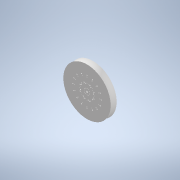
# Autodesk Inventor part: CenterIndexerWheel
Saved by Autodesk Inventor 2020 (Build 240168000, 168)
## iProperties
Created: 2020-01-19
Part Number: CenterIndexerWheel
Material: Generic
Document SubType Name: Modeling
Designer: srini
Density: 1 g/cm^3
Appearance: Default
Author: srini
Autodesk Inventor part; units mm, degrees
ref_plane "YZ Plane" through (0, 0, 0) normal (1, 0, 0) x (0, 1, 0)
ref_plane "XZ Plane" through (0, 0, 0) normal (0, 1, 0) x (-1, 0, 0)
ref_plane "XY Plane" through (0, 0, 0) normal (0, 0, 1) x (1, 0, 0)
sketch "Sketch1" plane through (0, 0, 0) normal (0, 0, 1) x (1, 0, 0)
  circle A0 centre (0, 0) radius 203.2
  dimension "d0" = 406.4
  constraints: 1 centre point, 1 coincident
  measures "d0" diameter of A0
extrude "Extrusion1" add sketch "Sketch1" along normal blind 50.8
sketch "Sketch2" plane through (0, 0, 0) normal (1, 0, 0) x (0, 1, 0)
  circle A0 centre (-285.75, 25.4) radius 88.9
  line L0 (203.2, 0) -> (-203.2, 0) projected
  line L1 (0, 149.86) -> (0, -99.06) projected
  point P0 (0, 0)
  dimension "d3" = 25.4
  dimension "d4" = 177.8
  dimension "d5" = 285.75
  constraints: 1 centre point
  measures "d3" distance from line of L0 A0.centre
  measures "d4" diameter of A0
  measures "d5" distance from line of L1 A0.centre
revolve "Revolution1" cut sketch "Sketch2" angle 360 about axis through (0, 0, 0) along (0, 0, -1)
sketch "Sketch3" plane through (0, 0, 0) normal (0, 0, -1) x (-1, 0, 0)
  point P0 (0, 0)
sketch "Sketch4" plane through (0, 0, 50.8) normal (0, 0, 1) x (1, 0, 0)
  line L0 (-3.6662, 6.35) -> (3.6662, 6.35)
  line L1 (3.6662, 6.35) -> (7.3323, 0)
  line L2 (7.3323, 0) -> (3.6662, -6.35)
  line L3 (3.6662, -6.35) -> (-3.6662, -6.35)
  line L4 (-3.6662, -6.35) -> (-7.3323, 0)
  line L5 (-7.3323, 0) -> (-3.6662, 6.35)
  circle A0 centre (0, 23.8125) radius 2.5797
  circle A1 centre (-11.9062, 20.6222) radius 2.5797
  circle A2 centre (-20.6222, 11.9063) radius 2.5797
  circle A3 centre (-23.8125, 0) radius 2.5797
  circle A4 centre (-20.6222, -11.9062) radius 2.5797
  circle A5 centre (-11.9063, -20.6222) radius 2.5797
  circle A6 centre (0, -23.8125) radius 2.5797
  circle A7 centre (11.9062, -20.6222) radius 2.5797
  circle A8 centre (20.6222, -11.9063) radius 2.5797
  circle A9 centre (23.8125, 0) radius 2.5797
  circle A10 centre (20.6222, 11.9062) radius 2.5797
  circle A11 centre (11.9063, 20.6222) radius 2.5797
  point P0 (0, 0)
  point P1 (0, 0)
  dimension "d7" = 12.7
  dimension "d8" = 23.8125
  dimension "d9" = 5.1594
  dimension "d12" = 360
  constraints: 12 centre point, 12 end point, 1 coincident, 1 horizontal, 1 vertical alignment, 38 other
  measures "d7" distance between parallel lines of L3 L0
  measures "d8" distance of point (0, 0) A0.centre
  measures "d9" diameter of A0
extrude "Extrusion2" cut sketch "Sketch4" against normal through all
sketch "Sketch6" plane through (0, 0, 0) normal (0, 0, -1) x (-1, 0, 0)
  circle A0 centre (0, 107.95) radius 2.5797
  circle A1 centre (0, 120.269) radius 4.445
  circle A2 centre (-41.3107, 99.7328) radius 2.5797
  circle A3 centre (-46.025, 111.1141) radius 4.445
  circle A4 centre (-76.3322, 76.3322) radius 2.5797
  circle A5 centre (-85.043, 85.043) radius 4.445
  circle A6 centre (-99.7328, 41.3107) radius 2.5797
  circle A7 centre (-111.1141, 46.025) radius 4.445
  circle A8 centre (-107.95, 0) radius 2.5797
  circle A9 centre (-120.269, 0) radius 4.445
  circle A10 centre (-99.7328, -41.3107) radius 2.5797
  circle A11 centre (-111.1141, -46.025) radius 4.445
  circle A12 centre (-76.3322, -76.3322) radius 2.5797
  circle A13 centre (-85.043, -85.043) radius 4.445
  circle A14 centre (-41.3107, -99.7328) radius 2.5797
  circle A15 centre (-46.025, -111.1141) radius 4.445
  circle A16 centre (0, -107.95) radius 2.5797
  circle A17 centre (0, -120.269) radius 4.445
  circle A18 centre (41.3107, -99.7328) radius 2.5797
  circle A19 centre (46.025, -111.1141) radius 4.445
  circle A20 centre (76.3322, -76.3322) radius 2.5797
  circle A21 centre (85.043, -85.043) radius 4.445
  circle A22 centre (99.7328, -41.3107) radius 2.5797
  circle A23 centre (111.1141, -46.025) radius 4.445
  circle A24 centre (107.95, 0) radius 2.5797
  circle A25 centre (120.269, 0) radius 4.445
  circle A26 centre (99.7328, 41.3107) radius 2.5797
  circle A27 centre (111.1141, 46.025) radius 4.445
  circle A28 centre (76.3322, 76.3322) radius 2.5797
  circle A29 centre (85.043, 85.043) radius 4.445
  circle A30 centre (41.3107, 99.7328) radius 2.5797
  circle A31 centre (46.025, 111.1141) radius 4.445
  point P0 (0, 0)
  dimension "d16" = 5.1594
  dimension "d17" = 107.95
  dimension "d18" = 8.89
  dimension "d19" = 120.269
  dimension "d22" = 360
  constraints: 32 centre point, 2 vertical alignment, 65 other
  measures "d16" diameter of A0
  measures "d17" distance of point (0, 0) A0.centre
  measures "d18" diameter of A1
  measures "d19" distance of point (0, 0) A1.centre
extrude "Extrusion3" cut sketch "Sketch6" against normal through all
sketch "Sketch7" plane through (0, 0, 50.8) normal (0, 0, 1) x (1, 0, 0)
  circle A0 centre (0, 63.4238) radius 2.032
  circle A1 centre (-44.8474, 44.8474) radius 2.032
  circle A2 centre (-63.4238, 0) radius 2.032
  circle A3 centre (-44.8474, -44.8474) radius 2.032
  circle A4 centre (0, -63.4238) radius 2.032
  circle A5 centre (44.8474, -44.8474) radius 2.032
  circle A6 centre (63.4238, 0) radius 2.032
  circle A7 centre (44.8474, 44.8474) radius 2.032
  line L0 (0, 63.4238) -> (0, 0) construction
  circle A8 centre (11.1717, 56.164) radius 2.032
  line L1 (11.1717, 56.164) -> (0, 0) construction
  circle A9 centre (24.2712, 58.596) radius 4.445
  line L2 (24.2712, 58.596) -> (0, 0) construction
  circle A10 centre (-24.2712, 58.596) radius 4.445
  circle A11 centre (-58.596, 24.2712) radius 4.445
  circle A12 centre (-58.596, -24.2712) radius 4.445
  circle A13 centre (-24.2712, -58.596) radius 4.445
  circle A14 centre (24.2712, -58.596) radius 4.445
  circle A15 centre (58.596, -24.2712) radius 4.445
  circle A16 centre (58.596, 24.2712) radius 4.445
  circle A17 centre (-31.8143, 47.6135) radius 2.032
  circle A18 centre (-56.164, 11.1717) radius 2.032
  circle A19 centre (-47.6135, -31.8143) radius 2.032
  circle A20 centre (-11.1717, -56.164) radius 2.032
  circle A21 centre (31.8143, -47.6135) radius 2.032
  circle A22 centre (56.164, -11.1717) radius 2.032
  circle A23 centre (47.6135, 31.8143) radius 2.032
  line L3 (31.8143, 47.6135) -> (0, 0) construction
  circle A24 centre (31.8143, 47.6135) radius 4.445
  circle A25 centre (-11.1717, 56.164) radius 4.445
  circle A26 centre (-47.6135, 31.8143) radius 4.445
  circle A27 centre (-56.164, -11.1717) radius 4.445
  circle A28 centre (-31.8143, -47.6135) radius 4.445
  circle A29 centre (11.1717, -56.164) radius 4.445
  circle A30 centre (47.6135, -31.8143) radius 4.445
  circle A31 centre (56.164, 11.1717) radius 4.445
  dimension "d26" = 4.064
  dimension "d27" = 63.4238
  dimension "d30" = 360
  dimension "d32" = 4.064
  dimension "d33" = 57.2643
  dimension "d34" = 11.25
  dimension "d35" = 8.89
  dimension "d36" = 22.5
  dimension "d39" = 360
  dimension "d43" = 360
  dimension "d45" = 33.75
  dimension "d48" = 360
  constraints: 32 centre point, 8 end point, 2 equal length, 1 coincident, 1 equal radius, 1 vertical, 1 vertical alignment, 68 other
  measures "d26" diameter of A0
  measures "d27" distance of L0.end L0.start
  measures "d32" diameter of A8
  measures "d33" distance of L1.start L0.end
  measures "d34" angle of L1 L0
  measures "d35" diameter of A9
  measures "d36" angle of L2 L0
  measures "d45" angle of L3 L0
extrude "Extrusion4" cut sketch "Sketch7" against normal through all
body "Solid1"
